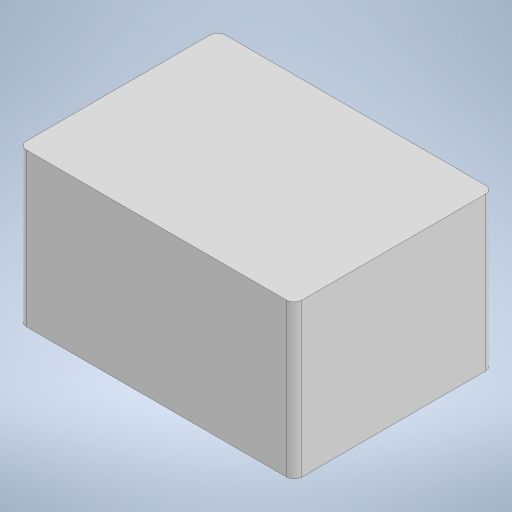
# Autodesk Inventor part: dxf
Saved by Autodesk Inventor 2023.2 (Build 272271000, 271)
## iProperties
Created: 2023-08-28
Part Number: dxf
Material: Generic
Document SubType Name: Modeling
Designer: yiako
Density: 1 g/cm^3
Appearance: Default
Author: yiako
Autodesk Inventor part; units mm, degrees
ref_plane "YZ Plane" through (0, 0, 0) normal (1, 0, 0) x (0, 1, 0)
ref_plane "XZ Plane" through (0, 0, 0) normal (0, 1, 0) x (-1, 0, 0)
ref_plane "XY Plane" through (0, 0, 0) normal (0, 0, 1) x (1, 0, 0)
sketch "Sketch1" plane through (0, 0, 0) normal (0, 1, 0) x (-1, 0, 0)
  line L0 (0.5, 0) -> (17.5, 0)
  line L1 (18, -0.5) -> (18, -12.5)
  line L2 (17.5, -13) -> (0.5, -13)
  line L3 (0, -12.5) -> (0, -0.5)
  arc A0 (18, -0.5) -> (17.5, 0) centre (17.5, -0.5) ccw
  arc A1 (17.5, -13) -> (18, -12.5) centre (17.5, -12.5) ccw
  arc A2 (0, -12.5) -> (0.5, -13) centre (0.5, -12.5) ccw
  arc A3 (0.5, 0) -> (0, -0.5) centre (0.5, -0.5) ccw
  point P0 (0, 0)
  point P1 (18, -13)
  point P2 (18, 0)
  point P3 (0, -13)
  dimension "d0" = 18
  dimension "d1" = 13
  dimension "d2" = 0.5
  constraints: 8 end point, 8 point on circle, 8 point on line, 8 tangent, 4 centre point, 3 equal radius, 2 parallel, 1 horizontal, 1 perpendicular
  measures "d0" distance of point (18, -13) point (0, -13)
  measures "d1" distance of point (18, 0) point (18, -13)
  measures "d2" radius of A0
extrude "Extrusion1" add sketch "Sketch1" along normal blind 10
body "Solid1"
